Autodesk Fusion 360 part; units mm, degrees
note: some values were not read from the file. Set by a fixed rule: which face or edge a step refers to.
(part 3 of 4)
sketch "Sketch60" plane through (0, 0, 0) normal (0, -1, 0) x (1, 0, 0)
  arc A0 (-197.8622, -246.9544) -> (-202.8622, -246.9544) centre (-200.3622, -246.9544) ccw
  line L0 (-197.8622, -246.9544) -> (-197.8622, -256.8986)
  line L1 (-197.8622, -256.8986) -> (-177.6941, -256.8986)
  line L2 (-177.6941, -256.8986) -> (-177.6941, -247.1839)
  arc A1 (-172.6941, -247.1839) -> (-177.6941, -247.1839) centre (-175.1941, -247.1839) ccw
  line L3 (-172.6941, -247.1839) -> (-142.6941, -247.1839)
  line L4 (-142.6941, -247.1839) -> (-142.6941, -154.3986)
  arc A2 (-142.6941, -149.3986) -> (-142.6941, -154.3986) centre (-142.6941, -151.8986) ccw
  line L5 (-142.6941, -149.3986) -> (-132.6941, -149.3986)
  line L6 (-132.6941, -149.3986) -> (-132.6941, -119.3986)
  line L7 (-132.6941, -119.3986) -> (-142.6941, -119.3986)
  arc A3 (-142.6941, -114.3986) -> (-142.6941, -119.3986) centre (-142.6941, -116.8986) ccw
  line L8 (-142.6941, -114.3986) -> (-142.6941, -16.8986)
  arc A4 (-142.6941, -11.8986) -> (-142.6941, -16.8986) centre (-142.6941, -14.3986) ccw
  line L9 (-142.6941, -11.8986) -> (-132.6941, -11.8986)
  line L10 (-132.6941, -11.8986) -> (-132.6941, 18.1014)
  line L11 (-132.6941, 18.1014) -> (-142.6941, 18.1014)
  arc A5 (-142.6941, 23.1014) -> (-142.6941, 18.1014) centre (-142.6941, 20.6014) ccw
  line L12 (-142.6941, 23.1014) -> (-142.6941, 120.6018)
  arc A6 (-142.6941, 125.6009) -> (-142.6941, 120.6018) centre (-142.6471, 123.1014) ccw
  line L13 (-142.6941, 125.6009) -> (-142.6941, 125.6014)
  line L14 (-142.6941, 125.6014) -> (-132.6941, 125.6014)
  line L15 (-132.6941, 125.6014) -> (-132.6941, 155.5705)
  line L16 (-132.6941, 155.5705) -> (-142.6941, 155.5705)
  line L17 (-142.6941, 155.5705) -> (-142.6941, 155.6018)
  arc A7 (-142.6941, 160.6009) -> (-142.6941, 155.6018) centre (-142.6471, 158.1014) ccw
  line L18 (-142.6941, 160.6009) -> (-142.6941, 263.1014)
  line L19 (-142.6941, 263.1014) -> (-167.6941, 263.1014)
  arc A8 (-172.6941, 263.1014) -> (-167.6941, 263.1014) centre (-170.1941, 263.1014) ccw
  line L20 (-172.6941, 263.1014) -> (-172.6941, 273.1014)
  line L21 (-172.6941, 273.1014) -> (-202.6941, 273.1014)
  line L22 (-202.6941, 273.1014) -> (-202.6941, 263.1014)
  arc A9 (-207.6941, 263.1014) -> (-202.6941, 263.1014) centre (-205.1941, 263.1014) ccw
  line L23 (-207.6941, 263.1014) -> (-232.6941, 263.1014)
  line L24 (-232.6941, 263.1014) -> (-232.6941, 198.1014)
  line L25 (-232.6941, 198.1014) -> (-222.6941, 198.1014)
  arc A10 (-222.6941, 193.1014) -> (-222.6941, 198.1014) centre (-222.6941, 195.6014) ccw
  line L26 (-222.6941, 193.1014) -> (-222.6941, 183.1014)
  arc A11 (-222.6941, 178.1014) -> (-222.6941, 183.1014) centre (-222.6941, 180.6014) ccw
  line L27 (-222.6941, 178.1014) -> (-232.6941, 178.1014)
  line L28 (-232.6941, 178.1014) -> (-232.6941, 163.1014)
  line L29 (-232.6941, 163.1014) -> (-332.6941, 163.1014)
  line L30 (-332.6941, 163.1014) -> (-332.6941, 178.1014)
  line L31 (-332.6941, 178.1014) -> (-342.6941, 178.1014)
  arc A12 (-342.6941, 183.1014) -> (-342.6941, 178.1014) centre (-342.6941, 180.6014) ccw
  line L32 (-342.6941, 183.1014) -> (-342.6941, 193.1014)
  arc A13 (-342.6941, 198.1014) -> (-342.6941, 193.1014) centre (-342.6941, 195.6014) ccw
  line L33 (-342.6941, 198.1014) -> (-332.6941, 198.1014)
  line L34 (-332.6941, 198.1014) -> (-332.6941, 263.1014)
  line L35 (-332.6941, 263.1014) -> (-357.6941, 263.1014)
  arc A14 (-362.6941, 263.1014) -> (-357.6941, 263.1014) centre (-360.1941, 263.1014) ccw
  line L36 (-362.6941, 263.1014) -> (-362.6941, 273.1014)
  line L37 (-362.6941, 273.1014) -> (-392.6941, 273.1014)
  line L38 (-392.6941, 273.1014) -> (-392.6941, 263.1014)
  arc A15 (-397.6941, 263.1014) -> (-392.6941, 263.1014) centre (-395.1941, 263.1014) ccw
  line L39 (-397.6941, 263.1014) -> (-422.6941, 263.1014)
  line L40 (-422.6941, 263.1014) -> (-422.6941, 160.6014)
  arc A16 (-422.6941, 155.6014) -> (-422.6941, 160.6014) centre (-422.6941, 158.1014) ccw
  line L41 (-422.6941, 155.6014) -> (-432.6941, 155.6014)
  line L42 (-432.6941, 155.6014) -> (-432.6941, 125.6014)
  line L43 (-432.6941, 125.6014) -> (-422.8505, 125.6014)
  arc A17 (-422.6941, 120.6038) -> (-422.8505, 125.6014) centre (-422.7723, 123.1026) ccw
  line L44 (-422.6941, 120.6038) -> (-422.6941, 23.1014)
  arc A18 (-422.6941, 18.1014) -> (-422.6941, 23.1014) centre (-422.6941, 20.6014) ccw
  line L45 (-422.6941, 18.1014) -> (-432.6941, 18.1014)
  line L46 (-432.6941, 18.1014) -> (-432.6941, -11.8986)
  line L47 (-432.6941, -11.8986) -> (-422.6941, -11.8986)
  arc A19 (-422.6941, -16.8986) -> (-422.6941, -11.8986) centre (-422.6941, -14.3986) ccw
  line L48 (-422.6941, -16.8986) -> (-422.6941, -114.3986)
  arc A20 (-422.6941, -119.3986) -> (-422.6941, -114.3986) centre (-422.6941, -116.8986) ccw
  line L49 (-422.6941, -119.3986) -> (-432.6941, -119.3986)
  line L50 (-432.6941, -119.3986) -> (-432.6941, -149.3986)
  line L51 (-432.6941, -149.3986) -> (-422.6941, -149.3986)
  arc A21 (-422.6941, -154.3986) -> (-422.6941, -149.3986) centre (-422.6941, -151.8986) ccw
  line L52 (-422.6941, -154.3986) -> (-422.6941, -246.8986)
  line L53 (-422.6941, -246.8986) -> (-392.6941, -246.8986)
  arc A22 (-387.6941, -246.8986) -> (-392.6941, -246.8986) centre (-390.1941, -246.8986) ccw
  line L54 (-387.6941, -246.8986) -> (-387.6941, -256.8986)
  line L55 (-387.6941, -256.8986) -> (-367.8622, -256.8986)
  line L56 (-367.8622, -256.8986) -> (-367.8622, -246.9544)
  arc A23 (-362.8622, -246.9544) -> (-367.8622, -246.9544) centre (-365.3622, -246.9544) ccw
  line L57 (-362.8622, -246.9544) -> (-202.8622, -246.9544)
  line L58 (-365.1941, -66.8986) -> (-365.1941, 98.1014)
  line L59 (-365.1941, 98.1014) -> (-200.1941, 98.1014)
  line L60 (-200.1941, 98.1014) -> (-200.1941, -66.8986)
  line L61 (-200.1941, -66.8986) -> (-365.1941, -66.8986)
  line L62 (-406.2361, -111.2993) -> (-206.2361, -111.2993)
  line L63 (-206.2361, -111.2993) -> (-206.2361, -161.2993)
  line L64 (-206.2361, -161.2993) -> (-406.2361, -161.2993)
  line L65 (-406.2361, -161.2993) -> (-406.2361, -111.2993)
  dimension "d334" = 200
  dimension "d335" = 50
  constraint horizontal L62
  constraint vertical L63
  constraint horizontal L64
  constraint vertical L65
  measures "d334" distance of L62.start L62.end
  measures "d335" distance of L62.start L64.end
extrude "Extrude39" add sketch "Sketch60" along normal blind 8 separate body contours L62 L63 L64 L65 makes body 10
sketch "Sketch61" plane through (-206.2361, 0, 0) normal (1, 0, 0) x (0, 1, 0)
  line L0 (0, -161.2993) -> (0, -111.2993)
  line L1 (0, -111.2993) -> (-8, -111.2993)
  line L2 (-8, -111.2993) -> (-8, -161.2993)
  line L3 (-8, -161.2993) -> (0, -161.2993)
  line L4 (-68, -111.2993) -> (-8, -111.2993)
  line L5 (-8, -111.2993) -> (-8, -161.2993)
  line L6 (-8, -161.2993) -> (-68, -161.2993)
  line L7 (-73, -156.2993) -> (-73, -116.2993)
  arc A0 (-68, -111.2993) -> (-73, -116.2993) centre (-68, -116.2993) ccw
  arc A1 (-73, -156.2993) -> (-68, -161.2993) centre (-68, -156.2993) ccw
  dimension "d340" = 10
  dimension "d341" = 10
  constraint horizontal L4
  constraint vertical L5
  constraint horizontal L6
  constraint vertical L7
  constraint coincident L1.end L2.start
  constraint tangent L4 A0
  constraint tangent L7 A0
  constraint tangent L6 A1
  constraint tangent L7 A1
  measures "d340" diameter of A0
  measures "d341" diameter of A1
extrude "Extrude40" add sketch "Sketch61" against normal blind 10 separate body contours L2 L4 L5 L6 L7 A0 A1 makes body 11
sketch "Sketch62" plane through (0, 0, 0) normal (0, 1, 0) x (1, 0, 0)
sketch "Sketch63" plane through (-216.2361, 0, 0) normal (-1, 0, 0) x (0, -1, 0)
  arc A0 (73, -116.2993) -> (68, -111.2993) centre (68, -116.2993) ccw
  line L0 (68, -111.2993) -> (8, -111.2993)
  line L1 (8, -111.2993) -> (8, -161.2993)
  line L2 (8, -161.2993) -> (68, -161.2993)
  arc A1 (68, -161.2993) -> (73, -156.2993) centre (68, -156.2993) ccw
  line L3 (73, -156.2993) -> (73, -116.2993)
  circle A2 centre (170, -90) radius 18.5
  dimension "d351" = 37
  measures "d351" diameter of A2
extrude "Extrude41" add sketch "Sketch63" along normal blind 57 separate body contours A2 makes body 12
sketch "Sketch64" plane through (-216.2361, 0, 0) normal (1, 0, 0) x (0, 1, 0)
  circle A0 centre (-170, -90) radius 3
  circle A1 centre (-170, -90) radius 18.5
  dimension "d357" = 6
  constraint concentric A0 A1
  measures "d357" diameter of A0
extrude "Extrude42" add sketch "Sketch64" along normal blind 20 contours A0 bodies 12
sketch "Sketch65" plane through (0, 0, -111.2993) normal (0, 0, 1) x (-1, 0, 0)
  line L0 (206.2361, 0) -> (406.2361, 0)
  line L1 (406.2361, 0) -> (406.2361, 8)
  line L2 (406.2361, 8) -> (206.2361, 8)
  line L3 (206.2361, 8) -> (206.2361, 0)
  line L4 (538, -190) -> (498, -190)
  line L5 (498, -190) -> (498, -188)
  line L6 (498, -188) -> (538, -188)
  line L7 (538, -188) -> (538, -190)
  line L8 (500, -190) -> (498, -190)
  line L9 (498, -190) -> (498, -147)
  line L10 (498, -147) -> (500, -147)
  line L11 (500, -147) -> (500, -190)
  dimension "d360" = 40
  dimension "d361" = 2
  dimension "d362" = 2
  dimension "d363" = 43
  constraint horizontal L4
  constraint vertical L5
  constraint horizontal L6
  constraint vertical L7
  constraint horizontal L8
  constraint vertical L9
  constraint horizontal L10
  constraint vertical L11
  constraint coincident L4.end L5.start
  measures "d360" distance of L4.start L4.end
  measures "d361" distance of L4.start L6.end
  measures "d362" distance of L8.start L4.end
  measures "d363" distance of L8.start L10.end
extrude "Extrude43" add sketch "Sketch65" along normal blind 40 separate body contours L4 L6 L7 L11 | L4 L5 L6 L8 L9 L11 | L6 L9 L10 L11 makes body 13
sketch "Sketch66" plane through (0, 0, 0) normal (0, 0, 1) x (1, 0, 0)
sketch "Sketch67" plane through (0, 0, 0) normal (0, -1, 0) x (1, 0, 0)
move_body "Move6" bodies 13 to x (1, 0, 0) y (0, 1, 0) z (0, 0, 1) at (-242.0057, 0, -461.3258)
sketch "Sketch68" plane through (-740.0057, 0, 0) normal (1, 0, 0) x (0, 1, 0)
  line L0 (147, -572.6251) -> (190, -572.6251)
  line L1 (190, -572.6251) -> (190, -532.6251)
  line L2 (190, -532.6251) -> (147, -532.6251)
  line L3 (147, -532.6251) -> (147, -572.6251)
  line L4 (167, -532.6251) -> (190, -532.6251)
  line L5 (190, -532.6251) -> (190, -572.6251)
  line L6 (190, -572.6251) -> (167, -572.6251)
  arc A0 (167, -532.6251) -> (167, -572.6251) centre (167, -552.6251) ccw
  dimension "d366" = 43
  constraint horizontal L4
  constraint vertical L5
  constraint horizontal L6
  constraint tangent L4 A0
  constraint tangent L6 A0
  measures "d366" distance of L2.end L1.end
extrude "Extrude44" cut sketch "Sketch68" against normal blind 2 contours L0 L3 A0 | L2 L3 A0 bodies 13
sketch "Sketch69" plane through (-740.0057, 0, 0) normal (1, 0, 0) x (0, 1, 0)
  arc A0 (167, -532.6251) -> (167, -572.6251) centre (167, -552.6251) ccw
  line L0 (167, -572.6251) -> (190, -572.6251)
  line L1 (190, -572.6251) -> (190, -532.6251)
  line L2 (190, -532.6251) -> (167, -532.6251)
  circle A1 centre (168.5, -552.6251) radius 3
  dimension "d370" = 6
  measures "d370" diameter of A1
extrude "Extrude45" cut sketch "Sketch69" against normal blind 2 contours A1 bodies 13
sketch "Sketch70" plane through (-742.0057, 0, 0) normal (-1, 0, 0) x (0, -1, 0)
  circle A0 centre (-168.5, -552.6251) radius 3
move_body "Move7" bodies 12 to x (1, 0, 0) y (0, 1, 0) z (0, 0, 1) at (0, -222.4188, 95.0256)
move_body "Move8" bodies 12 to x (1, 0, 0) y (0, 1, 0) z (0, 0, 1) at (-545, 614.0985, -612.4606)
move_body "Move9" bodies 12 to x (1, 0, 0) y (0, 0.965926, 0.258819) z (0, -0.258819, 0.965926) at (19.4785, -202.815, -23.1256)
move_body "Move10" bodies 12 13 to x (1, 0, 0) y (0, 1, 0) z (0, 0, 1) at (392.4146, -197.9462, 415.5182)
sketch "Sketch71" plane through (-347.591, 0, 0) normal (1, 0, 0) x (0, 1, 0)
  circle A0 centre (-29.4462, -137.1069) radius 3
  arc A1 (-30.9462, -117.1069) -> (-30.9462, -157.1069) centre (-30.9462, -137.1069) ccw
  line L0 (-30.9462, -157.1069) -> (-7.9462, -157.1069)
  line L1 (-7.9462, -157.1069) -> (-7.9462, -117.1069)
  line L2 (-7.9462, -117.1069) -> (-30.9462, -117.1069)
  circle A2 centre (-29.4462, -137.1069) radius 3
  dimension "d373" = 6
  constraint concentric A0 A2
  measures "d373" diameter of A2
extrude "Extrude46" add 1 faces at (-329.343, -30.6538, -136.491) along direction (1, 0, 0) blind 120 separate body on bodies 12 makes body 14
sketch "Sketch72" plane through (0, 0, 0) normal (0, 1, 0) x (1, 0, 0)
extrude "Extrude47" add 1 faces at (-209.343, -30.6538, -136.491) along direction (1, 0, 0) blind 10 on bodies 14 bodies 14
sketch "Sketch73" plane through (-206.2361, 0, 0) normal (1, 0, 0) x (0, 1, 0)
  arc A0 (-68, -111.2993) -> (-73, -116.2993) centre (-68, -116.2993) ccw
  line L0 (-73, -116.2993) -> (-73, -156.2993)
  arc A1 (-73, -156.2993) -> (-68, -161.2993) centre (-68, -156.2993) ccw
  line L1 (-68, -161.2993) -> (-8, -161.2993)
  line L2 (-8, -161.2993) -> (-8, -111.2993)
  line L3 (-8, -111.2993) -> (-68, -111.2993)
  circle A2 centre (-29.4462, -137.1069) radius 3.25
  circle A3 centre (-29.4462, -137.1069) radius 3
  dimension "d379" = 6.5
  constraint concentric A2 A3
  measures "d379" diameter of A2
extrude "Extrude48" cut sketch "Sketch73" against normal through all contours A3 bodies 11
sketch "Sketch74" plane through (-206.2361, 0, 0) normal (1, 0, 0) x (0, 1, 0)
sketch "Sketch75" plane through (-216.2361, 0, 0) normal (-1, 0, 0) x (0, -1, 0)
sketch "Sketch76" plane through (-206.2361, 0, 0) normal (1, 0, 0) x (0, 1, 0)
sketch "Sketch77" plane through (-199.343, 0, 0) normal (1, 0, 0) x (0, 1, 0)
sketch "Sketch78" plane through (-216.2361, 0, 0) normal (-1, 0, 0) x (0, -1, 0)
sketch "Sketch79" plane through (-216.2361, -40.5, -136.2993) normal (-1, 0, 0) x (0, -1, 0)
sketch "Sketch80" plane through (-206.2361, 0, 0) normal (1, 0, 0) x (0, 1, 0)
  line L0 (-35, -130) -> (-21.0963, -130)
  line L1 (-21.0963, -130) -> (-21.0963, -147.7881)
  line L2 (-21.0963, -147.7881) -> (-35, -147.7881)
  line L3 (-35, -147.7881) -> (-35, -130)
  constraint horizontal L0
  constraint vertical L1
  constraint horizontal L2
  constraint vertical L3
extrude "Extrude50" add sketch "Sketch80" against normal blind 10 bodies 11
sketch "Sketch81" plane through (-206.2361, 0, 0) normal (1, 0, 0) x (0, 1, 0)
  line L0 (-32.4193, -136.2247) -> (-26.4193, -136.2247)
  circle A0 centre (-29.4193, -136.2247) radius 3.25
  dimension "d387" = 6.5
  constraint horizontal L0
  constraint midpoint L0 A0.centre
  measures "d387" diameter of A0
extrude "Extrude51" cut sketch "Sketch81" against normal blind 10 bodies 11
move_face "MoveFace1" by (1, 0, 0) 1 faces at (-199.343, -30.6538, -136.491) on bodies 14
move_face "MoveFace2" by (0, 0, 1.4691) 1 faces at (-329.343, -28.1848, -137.4483) on bodies 14
move_body "Move11" bodies 14 to x (1, 0, 0) y (0, 1, 0) z (0, 0, 1) at (0, 0, 0.5)
move_body "Move12" bodies 14 to x (1, 0, 0) y (0, 1, 0) z (0, 0, 1) at (0, 0, 0.25)
move_body "Move13" bodies 12 to x (1, 0, 0) y (0, 1, 0) z (0, 0, 1) at (0, 0, 0.75)
move_body "Move14" bodies 13 to x (1, 0, 0) y (0, 1, 0) z (0, 0, 1) at (0, 0, 0.75)
sketch "Sketch83" plane through (0, 0, 0) normal (0, 0, 1) x (1, 0, 0)
sketch "Sketch84" plane through (-206.2361, 0, 0) normal (1, 0, 0) x (0, 1, 0)
sketch "Sketch85" plane through (-206.2361, 0, 0) normal (1, 0, 0) x (0, 1, 0)
  line L0 (-53.5087, -133.0971) -> (-40.8265, -133.0836)
  line L1 (-53.5087, -139.0701) -> (-40.8265, -139.0836)
  arc A0 (-52.9462, -133.0965) -> (-52.9462, -139.0707) centre (-53.2243, -136.0836) ccw
  arc A1 (-40.8265, -139.0836) -> (-40.8265, -133.0836) centre (-40.8233, -136.0836) ccw
  dimension "d394" = 6
  dimension "d395" = 6
  constraint coincident L0.start A0
  constraint tangent L0 A1
  constraint coincident L1.start A0
  constraint tangent L1 A1
  constraint coincident L1 A0.end
  constraint coincident L0 A0.start
  measures "d394" diameter of A1
  measures "d395" diameter of A0
sketch "Sketch86" plane through (-216.2361, 0, 0) normal (-1, 0, 0) x (0, -1, 0)
sketch "Sketch87" plane through (-216.2361, 0, 0) normal (-1, 0, 0) x (0, -1, 0)
  circle A0 centre (29.4193, -136.2196) radius 6.5
  circle A1 centre (29.4193, -136.2196) radius 3
  dimension "d398" = 13
  constraint concentric A0 A1
  measures "d398" diameter of A0
extrude "Extrude52" cut sketch "Sketch85" against normal blind 10 contours L0 L1 A0 A1 bodies 11
extrude "Extrude53" add sketch "Sketch87" along normal blind 90 bodies 14
sketch "Sketch88" plane through (0, -73, 0) normal (0, -1, 0) x (1, 0, 0)
  line L0 (-206.2361, -156.2993) -> (-206.2361, -116.2993)
  line L1 (-206.2361, -116.2993) -> (-216.2361, -116.2993)
  line L2 (-216.2361, -116.2993) -> (-216.2361, -156.2993)
  line L3 (-216.2361, -156.2993) -> (-206.2361, -156.2993)
  circle A0 centre (-211.2361, -136.2993) radius 3
  dimension "d403" = 6
  measures "d403" diameter of A0
extrude "Extrude54" cut sketch "Sketch88" against normal blind 10 contours A0 bodies 11
copy_body "CopyPasteBodies4" bodies 11 makes body 15
move_body "Move15" bodies 15 to x (1, 0, 0) y (0, 1, 0) z (0, 0, 1) at (-91, 0, 0)
move_body "Move16" bodies 15 to x (1, 0, 0) y (0, 1, 0) z (0, 0, 1) at (-10, 0, 0)
sketch "Sketch89" plane through (0, -73, 0) normal (0, -1, 0) x (1, 0, 0)
  circle A0 centre (-312.2361, -136.2993) radius 3
  line L0 (-307.2361, -156.2993) -> (-307.2361, -116.2993)
  line L1 (-307.2361, -116.2993) -> (-317.2361, -116.2993)
  line L2 (-317.2361, -116.2993) -> (-317.2361, -156.2993)
  line L3 (-317.2361, -156.2993) -> (-307.2361, -156.2993)
  line L4 (-317.2361, -116.2993) -> (-307.2361, -116.2993)
  line L5 (-307.2361, -116.2993) -> (-307.2361, -156.2993)
  line L6 (-307.2361, -156.2993) -> (-317.2361, -156.2993)
  line L7 (-317.2361, -156.2993) -> (-317.2361, -116.2993)
  line L8 (-312.2361, -116.2993) -> (-312.2361, -156.2993)
  circle A1 centre (-312.2361, -123.7993) radius 2
  circle A2 centre (-312.2361, -148.7993) radius 2
  dimension "d406" = 10
  dimension "d407" = 40
  dimension "d410" = 4
  dimension "d411" = 4
  constraint horizontal L4
  constraint vertical L5
  constraint horizontal L6
  constraint vertical L7
  constraint coincident L1.end L2.start
  constraint midpoint L4 L8.start
  constraint midpoint L6 L8.end
  constraint coincident L8 A1.centre
  constraint coincident L8 A2.centre
  measures "d406" distance of L1.end L0.end
  measures "d407" distance of L1.end L2.end
  measures "d410" diameter of A1
  measures "d411" diameter of A2
extrude "Extrude55" add sketch "Sketch89" along normal blind 3 separate body contours A0 L0 L1 L3 L4 L5 L6 L8 A1 A2 | A0 L1 L2 L3 L4 L6 L7 L8 A1 A2 makes body 16
copy_body "CopyPasteBodies5" bodies 16 makes body 17
move_body "Move17" bodies 17 to x (1, 0, 0) y (0, 1, 0) z (0, 0, 1) at (92, 0, 0)
move_body "Move18" bodies 17 to x (1, 0, 0) y (0, 1, 0) z (0, 0, 1) at (9, 0, 0)
sketch "Sketch90" plane through (-216.2361, 0, 0) normal (-1, 0, 0) x (0, -1, 0)
sketch "Sketch91" plane through (-216.2361, 0, 0) normal (-1, 0, 0) x (0, -1, 0)
  circle A0 centre (49.2242, -136.0566) radius 3
  dimension "d416" = 6
  measures "d416" diameter of A0
sketch "Sketch92" plane through (-216.2361, 0, 0) normal (-1, 0, 0) x (0, -1, 0)
surface "Extrude56" add extruded along (-1, 0, 0) between 0 and -15 path "Sketch91" along A0 separate body makes body 18
sketch "Sketch93" plane through (-206.2361, 0, 0) normal (1, 0, 0) x (0, 1, 0)
  circle A0 centre (-49.2242, -136.0566) radius 3
  circle A1 centre (-49.2242, -136.0566) radius 3
  dimension "d424" = 6
  constraint concentric A0 A1
  measures "d424" diameter of A0
extrude "Extrude57" cut sketch "Sketch93" against normal blind 110 bodies 15
delete_face "SurfaceDeleteFace1" leaving the opening 1 faces at (-206.2361, -51.9886, -134.8913) on bodies 18
sketch "Sketch94" plane through (-206.2361, 0, 0) normal (1, 0, 0) x (0, 1, 0)
  circle A0 centre (-29.4193, -136.2196) radius 6.5
  circle A1 centre (-29.4193, -136.2196) radius 3
  circle A2 centre (-48.4163, -135.8821) radius 12.5
  circle A3 centre (-48.4163, -135.8821) radius 3
  dimension "d427" = 13
  dimension "d428" = 25
  dimension "d429" = 6
  constraint concentric A0 A1
  constraint tangent A0 A2
  constraint concentric A2 A3
  measures "d427" diameter of A0
  measures "d428" diameter of A2
  measures "d429" diameter of A3
extrude "Extrude58" add sketch "Sketch94" along normal blind 10 and the other way blind 120 separate body contours A3 makes body 19
sketch "Sketch95" plane through (-196.2361, 0, 0) normal (1, 0, 0) x (0, 1, 0)
  circle A0 centre (-48.4163, -135.8821) radius 3
  circle A1 centre (-48.4163, -135.8821) radius 12.5
  dimension "d434" = 25
  constraint concentric A0 A1
  measures "d434" diameter of A1
extrude "Extrude59" add sketch "Sketch95" against normal blind 10 separate body contours A0 | A1 makes body 20
move_face "MoveFace3" to x (1, 0, 0) y (0, 1, 0) z (0, 0, 1) at (10, 0, 0) 1 faces at (-202.9028, -35.9318, -136.5052) on bodies 20
move_body "Move19" bodies 20 to x (1, 0, 0) y (0, 1, 0) z (0, 0, 1) at (-20, 0, 0)
move_face "MoveFace4" to x (1, 0, 0) y (0, 1, 0) z (0, 0, 1) at (-80, 0, 0) 1 faces at (-222.9028, -35.9318, -136.5052) on bodies 20
copy_body "CopyPasteBodies6" bodies 20 makes body 21
move_body "Move20" bodies 21 to x (1, 0, 0) y (0, 1, 0) z (0, 0, 1) at (-80, 0, 0)
copy_body "CopyPasteBodies7" bodies 20 makes body 22
move_body "Move21" bodies 22 to x (1, 0, 0) y (0, 1, 0) z (0, 0, 1) at (-40, 0, 0)
copy_body "CopyPasteBodies8" bodies 20 makes body 23
move_body "Move22" bodies 23 to x (1, 0, 0) y (0, 1, 0) z (0, 0, 1) at (-20, 0, 0)
copy_body "CopyPasteBodies9" bodies 22 makes body 24
move_body "Move23" bodies 24 to x (1, 0, 0) y (0, 1, 0) z (0, 0, 1) at (-20, 0, 0)
move_body "Move24" bodies 9 to x (-0.707107, -0.707107, 0) y (0.707107, -0.707107, 0) z (0, 0, 1) at (-660.8733, -493.7427, 0)
sketch "Sketch96" plane through (0, -10, 0) normal (0, -1, 0) x (1, 0, 0)
  line L0 (-200.1941, -66.8986) -> (-365.1941, -66.8986)
  line L1 (-365.1941, -66.8986) -> (-365.1941, 98.1014)
  line L2 (-365.1941, 98.1014) -> (-200.1941, 98.1014)
  line L3 (-200.1941, 98.1014) -> (-200.1941, -66.8986)
  line L4 (-142.6941, 135.6014) -> (-422.6941, 135.6014)
  line L5 (-422.6941, 135.6014) -> (-422.6941, -104.3986)
  line L6 (-422.6941, -104.3986) -> (-142.6941, -104.3986)
  line L7 (-142.6941, -104.3986) -> (-142.6941, 135.6014)
  line L8 (-365.1941, 98.1014) -> (-200.1941, 98.1014)
  line L9 (-200.1941, 98.1014) -> (-200.1941, -66.8986)
  line L10 (-200.1941, -66.8986) -> (-365.1941, -66.8986)
  line L11 (-365.1941, -66.8986) -> (-365.1941, 98.1014)
  line L12 (-382.6941, 115.6014) -> (-182.6941, 115.6014)
  line L13 (-182.6941, 115.6014) -> (-182.6941, -84.3986)
  line L14 (-182.6941, -84.3986) -> (-382.6941, -84.3986)
  line L15 (-382.6941, -84.3986) -> (-382.6941, 115.6014)
  dimension "d438" = 165
  dimension "d439" = 165
  dimension "d440" = 200
  dimension "d441" = 200
  constraint horizontal L8
  constraint vertical L9
  constraint horizontal L10
  constraint vertical L11
  constraint coincident L1.end L2.start
  constraint horizontal L12
  constraint vertical L13
  constraint horizontal L14
  constraint vertical L15
  measures "d438" distance of L1.end L2.end
  measures "d439" distance of L1.end L0.end
  measures "d440" distance of L12.start L12.end
  measures "d441" distance of L12.start L14.end
extrude "Extrude60" add sketch "Sketch96" along normal blind 3 separate body contours L12 L13 L14 L15 makes body 25
sketch "Sketch97" plane through (0, -13, 0) normal (0, -1, 0) x (1, 0, 0)
  line L0 (-200.1941, -66.8986) -> (-365.1941, -66.8986)
  line L1 (-365.1941, -66.8986) -> (-365.1941, 98.1014)
  line L2 (-365.1941, 98.1014) -> (-200.1941, 98.1014)
  line L3 (-200.1941, 98.1014) -> (-200.1941, -66.8986)
  line L4 (-382.6941, -84.3986) -> (-182.6941, -84.3986)
  line L5 (-182.6941, -84.3986) -> (-182.6941, 115.6014)
  line L6 (-182.6941, 115.6014) -> (-382.6941, 115.6014)
  line L7 (-382.6941, 115.6014) -> (-382.6941, -84.3986)
  line L8 (-376.8614, -55.2314) -> (-353.5268, -78.5659)
  line L9 (-353.5268, -78.5659) -> (-360.5979, -85.637)
  line L10 (-360.5979, -85.637) -> (-383.9324, -62.3024)
  line L11 (-383.9324, -62.3024) -> (-376.8614, -55.2314)
  line L12 (-181.4558, 93.5052) -> (-188.5268, 86.4341)
  line L13 (-211.8614, 109.7686) -> (-204.7903, 116.8397)
  line L14 (-188.5268, 86.4341) -> (-211.8614, 109.7686)
  line L15 (-204.7903, 116.8397) -> (-181.4558, 93.5052)
  line L16 (-353.5268, 109.7686) -> (-376.8614, 86.4341)
  line L17 (-383.9324, 93.5052) -> (-360.5979, 116.8397)
  line L18 (-360.5979, 116.8397) -> (-353.5268, 109.7686)
  line L19 (-376.8614, 86.4341) -> (-383.9324, 93.5052)
  line L20 (-210.8007, -77.5052) -> (-189.5875, -56.292)
  line L21 (-189.5875, -56.292) -> (-182.5164, -63.3631)
  line L22 (-182.5164, -63.3631) -> (-203.7296, -84.5763)
  line L23 (-203.7296, -84.5763) -> (-210.8007, -77.5052)
  dimension "d444" = 33
  dimension "d445" = 10
  dimension "d446" = 33
  dimension "d447" = 10
  dimension "d448" = 33
  dimension "d449" = 10
  dimension "d450" = 30
  dimension "d451" = 10
  constraint midpoint L2.end L14
  constraint midpoint L0.end L8
  constraint midpoint L1.end L16
  constraint midpoint L0.start L20
  measures "d444" distance of L8.start L8.end
  measures "d445" distance of L8.start L10.end
  measures "d446" distance of L12.start L13.end
  measures "d447" distance of L13.end L13.start
  measures "d448" distance of L16.end L16.start
  measures "d449" distance of L16.start L17.end
  measures "d450" distance of L20.start L20.end
  measures "d451" distance of L20.start L22.end
extrude "Extrude61" add sketch "Sketch97" along normal blind 25 separate body contours L4 L5 L20 L21 L22 L23 | L4 L7 L8 L9 L10 L11 | L5 L6 L12 L13 L14 L15 | L6 L7 L16 L17 L18 L19 makes body 26 at (-196.305, -29.6667, 94.2123) makes body 27 at (-203.7296, -21.3333, -70.4342) makes body 28 at (-361.305, -29.6667, 101.9904) makes body 29 at (-369.0832, -21.3333, -63.0096)
sketch "Sketch98" plane through (0, 0, 0) normal (0, -1, 0) x (1, 0, 0)
  circle A0 centre (-282.6941, 15.6014) radius 82.5
  line L0 (-392.6941, 136.1014) -> (-172.6941, 136.1014)
  line L1 (-152.6941, 116.1014) -> (-152.6941, -83.8986)
  line L2 (-172.6941, -103.8986) -> (-392.6941, -103.8986)
  line L3 (-412.6941, -83.8986) -> (-412.6941, 116.1014)
  line L4 (-392.6941, 136.1014) -> (-412.6941, 116.1014)
  line L5 (-172.6941, 136.1014) -> (-152.6941, 116.1014)
  line L6 (-412.6941, -83.8986) -> (-392.6941, -103.8986)
  line L7 (-172.6941, -103.8986) -> (-152.6941, -83.8986)
  point P0 (-412.6941, 136.1014)
  point P1 (-152.6941, 136.1014)
  point P2 (-152.6941, -103.8986)
  point P3 (-412.6941, -103.8986)
  point P4 (-142.6941, 18.1014)
  dimension "d454" = 260
  dimension "d455" = 240
  dimension "d456" = 20
  dimension "d457" = 20
  dimension "d458" = 20
  dimension "d459" = 20
  dimension "d460" = 20
  dimension "d461" = 20
  dimension "d462" = 20
  dimension "d463" = 20
  constraint horizontal L0
  constraint vertical L1
  constraint horizontal L2
  constraint vertical L3
  constraint coincident P0 L0
  constraint coincident P0 L3
  constraint coincident P1 L0
  constraint coincident P1 L1
  constraint coincident P3 L3
  constraint coincident P3 L2
  constraint coincident P2 L2
  constraint coincident P2 L1
  measures "d454" distance of P0 P1
  measures "d455" distance of P0 P3
  measures "d456" distance of P0 L0.start
  measures "d457" distance of P0 L3.end
  measures "d458" distance of P1 L0.end
  measures "d459" distance of P1 L1.start
  measures "d460" distance of P3 L3.start
  measures "d461" distance of P3 L2.end
  measures "d462" distance of P2 L2.start
  measures "d463" distance of P2 L1.end
extrude "Extrude62" add sketch "Sketch98" along normal blind 3 separate body makes body 30
sketch "Sketch99" plane through (-132.6941, 0, 0) normal (1, 0, 0) x (0, 1, 0)
  circle A0 centre (-25, -180) radius 4
  circle A1 centre (-50, 175) radius 4
  circle A2 centre (-25, 170) radius 4
  circle A3 centre (-50, -175) radius 4
  circle A4 centre (-75, 180) radius 4
  circle A5 centre (-75, -170) radius 4
  line L0 (0, 130.6014) -> (0, 150.6014)
  arc A6 (0, 155.6014) -> (0, 150.6014) centre (0, 153.1014) ccw
  line L1 (0, 155.6014) -> (10, 155.6014)
  line L2 (10, 155.6014) -> (10, 273.6512)
  line L3 (10, 273.6512) -> (-30, 273.6512)
  line L4 (-30, 273.6512) -> (-30, 263.6512)
  arc A7 (-35, 263.6512) -> (-30, 263.6512) centre (-32.5, 263.6512) ccw
  line L5 (-35, 263.6512) -> (-55, 263.6512)
  arc A8 (-60, 263.6512) -> (-55, 263.6512) centre (-57.5, 263.6512) ccw
  line L6 (-60, 263.6512) -> (-60, 273.6512)
  line L7 (-60, 273.6512) -> (-100, 273.6512)
  line L8 (-100, 273.6512) -> (-100, -256.3488)
  line L9 (-100, -256.3488) -> (-60, -256.3488)
  line L10 (-60, -256.3488) -> (-60, -246.3488)
  arc A9 (-55, -246.3488) -> (-60, -246.3488) centre (-57.5, -246.3488) ccw
  line L11 (-55, -246.3488) -> (-35, -246.3488)
  arc A10 (-30, -246.3488) -> (-35, -246.3488) centre (-32.5, -246.3488) ccw
  line L12 (-30, -246.3488) -> (-30, -256.3488)
  line L13 (-30, -256.3488) -> (10, -256.3488)
  line L14 (10, -256.3488) -> (10, -149.3986)
  line L15 (10, -149.3986) -> (0, -149.3986)
  arc A11 (0, -144.3986) -> (0, -149.3986) centre (0, -146.8986) ccw
  line L16 (0, -144.3986) -> (0, -124.3986)
  arc A12 (0, -119.3986) -> (0, -124.3986) centre (0, -121.8986) ccw
  line L17 (0, -119.3986) -> (10, -119.3986)
  line L18 (10, -119.3986) -> (10, -11.8986)
  line L19 (10, -11.8986) -> (0, -11.8986)
  arc A13 (0, -6.8986) -> (0, -11.8986) centre (0, -9.3986) ccw
  line L20 (0, -6.8986) -> (0, 13.1014)
  arc A14 (0, 18.1014) -> (0, 13.1014) centre (0, 15.6014) ccw
  line L21 (0, 18.1014) -> (10, 18.1014)
  line L22 (10, 18.1014) -> (10, 125.6014)
  line L23 (10, 125.6014) -> (0, 125.6014)
  arc A15 (0, 130.6014) -> (0, 125.6014) centre (0, 128.1014) ccw
  circle A16 centre (-75, 160) radius 4
  circle A17 centre (-50, 155) radius 4
  circle A18 centre (-25, 150) radius 4
  circle A19 centre (-75, 140) radius 4
  circle A20 centre (-50, 135) radius 4
  circle A21 centre (-25, 130) radius 4
  circle A22 centre (-75, 120) radius 4
  circle A23 centre (-50, 115) radius 4
  circle A24 centre (-25, 110) radius 4
  dimension "d468" = 20
  dimension "d469" = 20
  dimension "d470" = 8
  dimension "d471" = 8
  dimension "d472" = 8
  dimension "d473" = 8
  dimension "d474" = 8
  dimension "d475" = 8
  dimension "d476" = 8
  dimension "d477" = 8
  dimension "d478" = 8
  measures "d468" distance of A4.centre A16.centre
  measures "d469" distance of A1.centre A17.centre
  measures "d470" diameter of A16
  measures "d471" diameter of A17
  measures "d472" diameter of A18
  measures "d473" diameter of A19
  measures "d474" diameter of A20
  measures "d475" diameter of A21
  measures "d476" diameter of A22
  measures "d477" diameter of A23
  measures "d478" diameter of A24
extrude "Extrude63" cut sketch "Sketch99" against normal blind 10 contours A16 | A17 | A18 | A19 | A20 | A21 | A22 | A23 | A24 bodies 2
sketch "Sketch100" plane through (-132.6941, 0, 0) normal (1, 0, 0) x (0, 1, 0)
  circle A0 centre (-75, 120) radius 4
  circle A1 centre (-25, 150) radius 4
  circle A2 centre (-50, 155) radius 4
  circle A3 centre (-25, 130) radius 4
  circle A4 centre (-50, 115) radius 4
  circle A5 centre (-75, 140) radius 4
  circle A6 centre (-75, 160) radius 4
  circle A7 centre (-50, 135) radius 4
  circle A8 centre (-25, 110) radius 4
  circle A9 centre (-25, -180) radius 4
  circle A10 centre (-50, 175) radius 4
  circle A11 centre (-25, 170) radius 4
  circle A12 centre (-50, -175) radius 4
  circle A13 centre (-75, 180) radius 4
  circle A14 centre (-75, -170) radius 4
  line L0 (0, 130.6014) -> (0, 150.6014)
  arc A15 (0, 155.6014) -> (0, 150.6014) centre (0, 153.1014) ccw
  line L1 (0, 155.6014) -> (10, 155.6014)
  line L2 (10, 155.6014) -> (10, 273.6512)
  line L3 (10, 273.6512) -> (-30, 273.6512)
  line L4 (-30, 273.6512) -> (-30, 263.6512)
  arc A16 (-35, 263.6512) -> (-30, 263.6512) centre (-32.5, 263.6512) ccw
  line L5 (-35, 263.6512) -> (-55, 263.6512)
  arc A17 (-60, 263.6512) -> (-55, 263.6512) centre (-57.5, 263.6512) ccw
  line L6 (-60, 263.6512) -> (-60, 273.6512)
  line L7 (-60, 273.6512) -> (-100, 273.6512)
  line L8 (-100, 273.6512) -> (-100, -256.3488)
  line L9 (-100, -256.3488) -> (-60, -256.3488)
  line L10 (-60, -256.3488) -> (-60, -246.3488)
  arc A18 (-55, -246.3488) -> (-60, -246.3488) centre (-57.5, -246.3488) ccw
  line L11 (-55, -246.3488) -> (-35, -246.3488)
  arc A19 (-30, -246.3488) -> (-35, -246.3488) centre (-32.5, -246.3488) ccw
  line L12 (-30, -246.3488) -> (-30, -256.3488)
  line L13 (-30, -256.3488) -> (10, -256.3488)
  line L14 (10, -256.3488) -> (10, -149.3986)
  line L15 (10, -149.3986) -> (0, -149.3986)
  arc A20 (0, -144.3986) -> (0, -149.3986) centre (0, -146.8986) ccw
  line L16 (0, -144.3986) -> (0, -124.3986)
  arc A21 (0, -119.3986) -> (0, -124.3986) centre (0, -121.8986) ccw
  line L17 (0, -119.3986) -> (10, -119.3986)
  line L18 (10, -119.3986) -> (10, -11.8986)
  line L19 (10, -11.8986) -> (0, -11.8986)
  arc A22 (0, -6.8986) -> (0, -11.8986) centre (0, -9.3986) ccw
  line L20 (0, -6.8986) -> (0, 13.1014)
  arc A23 (0, 18.1014) -> (0, 13.1014) centre (0, 15.6014) ccw
  line L21 (0, 18.1014) -> (10, 18.1014)
  line L22 (10, 18.1014) -> (10, 125.6014)
  line L23 (10, 125.6014) -> (0, 125.6014)
  arc A24 (0, 130.6014) -> (0, 125.6014) centre (0, 128.1014) ccw
  circle A25 centre (-75, 100) radius 4
  circle A26 centre (-50, 95) radius 4
  circle A27 centre (-25, 90) radius 4
  circle A28 centre (-75, 80) radius 4
  circle A29 centre (-50, 75) radius 4
  circle A30 centre (-25, 70) radius 4
  dimension "d481" = 8
  dimension "d482" = 8
  dimension "d483" = 8
  dimension "d484" = 8
  dimension "d485" = 8
  dimension "d486" = 8
  measures "d481" diameter of A25
  measures "d482" diameter of A26
  measures "d483" diameter of A27
  measures "d484" diameter of A28
  measures "d485" diameter of A29
  measures "d486" diameter of A30
extrude "Extrude64" cut sketch "Sketch100" against normal blind 10 contours A25 | A26 | A27 | A28 | A29 | A30 bodies 2
sketch "Sketch101" plane through (-132.6941, 0, 0) normal (1, 0, 0) x (0, 1, 0)
  circle A0 centre (-75, 80) radius 4
  circle A1 centre (-75, 100) radius 4
  circle A2 centre (-50, 75) radius 4
  circle A3 centre (-25, 90) radius 4
  circle A4 centre (-50, 95) radius 4
  circle A5 centre (-25, 70) radius 4
  circle A6 centre (-75, 120) radius 4
  circle A7 centre (-25, 150) radius 4
  circle A8 centre (-50, 155) radius 4
  circle A9 centre (-25, 130) radius 4
  circle A10 centre (-50, 115) radius 4
  circle A11 centre (-75, 140) radius 4
  circle A12 centre (-75, 160) radius 4
  circle A13 centre (-50, 135) radius 4
  circle A14 centre (-25, 110) radius 4
  circle A15 centre (-25, -180) radius 4
  circle A16 centre (-50, 175) radius 4
  circle A17 centre (-25, 170) radius 4
  circle A18 centre (-50, -175) radius 4
  circle A19 centre (-75, 180) radius 4
  circle A20 centre (-75, -170) radius 4
  line L0 (0, 130.6014) -> (0, 150.6014)
  arc A21 (0, 155.6014) -> (0, 150.6014) centre (0, 153.1014) ccw
  line L1 (0, 155.6014) -> (10, 155.6014)
  line L2 (10, 155.6014) -> (10, 273.6512)
  line L3 (10, 273.6512) -> (-30, 273.6512)
  line L4 (-30, 273.6512) -> (-30, 263.6512)
  arc A22 (-35, 263.6512) -> (-30, 263.6512) centre (-32.5, 263.6512) ccw
  line L5 (-35, 263.6512) -> (-55, 263.6512)
  arc A23 (-60, 263.6512) -> (-55, 263.6512) centre (-57.5, 263.6512) ccw
  line L6 (-60, 263.6512) -> (-60, 273.6512)
  line L7 (-60, 273.6512) -> (-100, 273.6512)
  line L8 (-100, 273.6512) -> (-100, -256.3488)
  line L9 (-100, -256.3488) -> (-60, -256.3488)
  line L10 (-60, -256.3488) -> (-60, -246.3488)
  arc A24 (-55, -246.3488) -> (-60, -246.3488) centre (-57.5, -246.3488) ccw
  line L11 (-55, -246.3488) -> (-35, -246.3488)
  arc A25 (-30, -246.3488) -> (-35, -246.3488) centre (-32.5, -246.3488) ccw
  line L12 (-30, -246.3488) -> (-30, -256.3488)
  line L13 (-30, -256.3488) -> (10, -256.3488)
  line L14 (10, -256.3488) -> (10, -149.3986)
  line L15 (10, -149.3986) -> (0, -149.3986)
  arc A26 (0, -144.3986) -> (0, -149.3986) centre (0, -146.8986) ccw
  line L16 (0, -144.3986) -> (0, -124.3986)
  arc A27 (0, -119.3986) -> (0, -124.3986) centre (0, -121.8986) ccw
  line L17 (0, -119.3986) -> (10, -119.3986)
  line L18 (10, -119.3986) -> (10, -11.8986)
  line L19 (10, -11.8986) -> (0, -11.8986)
  arc A28 (0, -6.8986) -> (0, -11.8986) centre (0, -9.3986) ccw
  line L20 (0, -6.8986) -> (0, 13.1014)
  arc A29 (0, 18.1014) -> (0, 13.1014) centre (0, 15.6014) ccw
  line L21 (0, 18.1014) -> (10, 18.1014)
  line L22 (10, 18.1014) -> (10, 125.6014)
  line L23 (10, 125.6014) -> (0, 125.6014)
  arc A30 (0, 130.6014) -> (0, 125.6014) centre (0, 128.1014) ccw
  circle A31 centre (-75, -150) radius 4
  circle A32 centre (-50, -155) radius 4
  circle A33 centre (-25, -160) radius 4
  circle A34 centre (-75, -130.3823) radius 4
  circle A35 centre (-50.7025, -135.281) radius 4
  circle A36 centre (-25, -140) radius 4
  circle A37 centre (-75, -110) radius 4
  circle A38 centre (-50, -115) radius 4
  circle A39 centre (-25, -120) radius 4
  circle A40 centre (-75, -90) radius 4
  circle A41 centre (-50, -95) radius 4
  circle A42 centre (-25, -100) radius 4
  circle A43 centre (-75, -70) radius 4
  circle A44 centre (-50, -75) radius 4
  circle A45 centre (-25, -80) radius 4
  dimension "d489" = 8
  dimension "d490" = 8
  dimension "d491" = 8
  dimension "d492" = 8
  dimension "d493" = 8
  dimension "d494" = 8
  dimension "d495" = 8
  dimension "d496" = 8
  dimension "d497" = 8
  dimension "d498" = 8
  dimension "d499" = 8
  dimension "d500" = 8
  dimension "d501" = 8
  dimension "d502" = 8
  dimension "d503" = 8
  measures "d489" diameter of A31
  measures "d490" diameter of A32
  measures "d491" diameter of A33
  measures "d492" diameter of A34
  measures "d493" diameter of A35
  measures "d494" diameter of A36
  measures "d495" diameter of A37
  measures "d496" diameter of A38
  measures "d497" diameter of A39
  measures "d498" diameter of A40
  measures "d499" diameter of A41
  measures "d500" diameter of A42
  measures "d501" diameter of A43
  measures "d502" diameter of A44
  measures "d503" diameter of A45
extrude "Extrude65" cut sketch "Sketch101" against normal blind 10 contours A31 | A32 | A33 | A34 | A35 | A36 | A37 | A38 | A39 | A40 | A41 | A42 | A43 | A44 | A45 bodies 2
sketch "Sketch102" plane through (-422.6941, 0, 0) normal (1, 0, 0) x (0, 1, 0)
  arc A0 (0, 130.6014) -> (0, 125.6014) centre (0, 128.1014) ccw
  line L0 (0, 130.6014) -> (0, 150.6014)
  arc A1 (0, 155.6014) -> (0, 150.6014) centre (0, 153.1014) ccw
  line L1 (0, 155.6014) -> (10, 155.6014)
  line L2 (10, 155.6014) -> (10, 273.6512)
  line L3 (10, 273.6512) -> (-30, 273.6512)
  line L4 (-30, 273.6512) -> (-30, 263.6512)
  arc A2 (-35, 263.6512) -> (-30, 263.6512) centre (-32.5, 263.6512) ccw
  line L5 (-35, 263.6512) -> (-55, 263.6512)
  arc A3 (-60, 263.6512) -> (-55, 263.6512) centre (-57.5, 263.6512) ccw
  line L6 (-60, 263.6512) -> (-60, 273.6512)
  line L7 (-60, 273.6512) -> (-100, 273.6512)
  line L8 (-100, 273.6512) -> (-100, -256.3488)
  line L9 (-100, -256.3488) -> (-60, -256.3488)
  line L10 (-60, -256.3488) -> (-60, -246.3488)
  arc A4 (-55, -246.3488) -> (-60, -246.3488) centre (-57.5, -246.3488) ccw
  line L11 (-55, -246.3488) -> (-35, -246.3488)
  arc A5 (-30, -246.3488) -> (-35, -246.3488) centre (-32.5, -246.3488) ccw
  line L12 (-30, -246.3488) -> (-30, -256.3488)
  line L13 (-30, -256.3488) -> (10, -256.3488)
  line L14 (10, -256.3488) -> (10, -149.3986)
  line L15 (10, -149.3986) -> (0, -149.3986)
  arc A6 (0, -144.3986) -> (0, -149.3986) centre (0, -146.8986) ccw
  line L16 (0, -144.3986) -> (0, -124.3986)
  arc A7 (0, -119.3986) -> (0, -124.3986) centre (0, -121.8986) ccw
  line L17 (0, -119.3986) -> (10, -119.3986)
  line L18 (10, -119.3986) -> (10, -11.8986)
  line L19 (10, -11.8986) -> (0, -11.8986)
  arc A8 (0, -6.8986) -> (0, -11.8986) centre (0, -9.3986) ccw
  line L20 (0, -6.8986) -> (0, 13.1014)
  arc A9 (0, 18.1014) -> (0, 13.1014) centre (0, 15.6014) ccw
  line L21 (0, 18.1014) -> (10, 18.1014)
  line L22 (10, 18.1014) -> (10, 125.6014)
  line L23 (10, 125.6014) -> (0, 125.6014)
  circle A10 centre (-25, -180) radius 4
  circle A11 centre (-50, 175) radius 4
  circle A12 centre (-25, 170) radius 4
  circle A13 centre (-50, -175) radius 4
  circle A14 centre (-75, 180) radius 4
  circle A15 centre (-75, -170) radius 4
  circle A16 centre (-75, 160) radius 4
  circle A17 centre (-50, 155) radius 4
  circle A18 centre (-25, 150) radius 4
  circle A19 centre (-75, 140) radius 4
  circle A20 centre (-50, 134) radius 4
  circle A21 centre (-25, 130) radius 4
  circle A22 centre (-75, 120) radius 4
  circle A23 centre (-50, 115) radius 4
  circle A24 centre (-25, 110) radius 4
  circle A25 centre (-75, 100) radius 4
  circle A26 centre (-50, 95) radius 4
  circle A27 centre (-25, 90) radius 4
  circle A28 centre (-75, 80) radius 4
  circle A29 centre (-50, 75) radius 4
  circle A30 centre (-25, 70) radius 4
  dimension "d506" = 20
  dimension "d507" = 8
  dimension "d508" = 8
  dimension "d509" = 8
  dimension "d510" = 8
  dimension "d511" = 8
  dimension "d512" = 8
  dimension "d513" = 8
  dimension "d514" = 8
  dimension "d515" = 8
  dimension "d516" = 8
  dimension "d517" = 8
  dimension "d518" = 8
  dimension "d519" = 8
  dimension "d520" = 8
  dimension "d521" = 8
  measures "d506" distance of A14.centre A16.centre
  measures "d507" diameter of A16
  measures "d508" diameter of A17
  measures "d509" diameter of A18
  measures "d510" diameter of A19
  measures "d511" diameter of A20
  measures "d512" diameter of A21
  measures "d513" diameter of A22
  measures "d514" diameter of A23
  measures "d515" diameter of A24
  measures "d516" diameter of A25
  measures "d517" diameter of A26
  measures "d518" diameter of A27
  measures "d519" diameter of A28
  measures "d520" diameter of A29
  measures "d521" diameter of A30
extrude "Extrude66" cut sketch "Sketch102" against normal blind 10 contours A16 | A17 | A18 | A19 | A20 | A21 | A22 | A23 | A24 | A25 | A26 | A27 | A28 | A29 | A30 bodies 3
sketch "Sketch103" plane through (-422.6941, 0, 0) normal (1, 0, 0) x (0, 1, 0)
  circle A0 centre (-75, 80) radius 4
  circle A1 centre (-25, 110) radius 4
  circle A2 centre (-50, 134) radius 4
  circle A3 centre (-75, 160) radius 4
  circle A4 centre (-75, 140) radius 4
  circle A5 centre (-50, 115) radius 4
  circle A6 centre (-25, 90) radius 4
  circle A7 centre (-50, 75) radius 4
  circle A8 centre (-75, 100) radius 4
  circle A9 centre (-25, 130) radius 4
  circle A10 centre (-50, 155) radius 4
  circle A11 centre (-25, 150) radius 4
  circle A12 centre (-75, 120) radius 4
  circle A13 centre (-50, 95) radius 4
  circle A14 centre (-25, 70) radius 4
  arc A15 (0, 130.6014) -> (0, 125.6014) centre (0, 128.1014) ccw
  line L0 (0, 130.6014) -> (0, 150.6014)
  arc A16 (0, 155.6014) -> (0, 150.6014) centre (0, 153.1014) ccw
  line L1 (0, 155.6014) -> (10, 155.6014)
  line L2 (10, 155.6014) -> (10, 273.6512)
  line L3 (10, 273.6512) -> (-30, 273.6512)
  line L4 (-30, 273.6512) -> (-30, 263.6512)
  arc A17 (-35, 263.6512) -> (-30, 263.6512) centre (-32.5, 263.6512) ccw
  line L5 (-35, 263.6512) -> (-55, 263.6512)
  arc A18 (-60, 263.6512) -> (-55, 263.6512) centre (-57.5, 263.6512) ccw
  line L6 (-60, 263.6512) -> (-60, 273.6512)
  line L7 (-60, 273.6512) -> (-100, 273.6512)
  line L8 (-100, 273.6512) -> (-100, -256.3488)
  line L9 (-100, -256.3488) -> (-60, -256.3488)
  line L10 (-60, -256.3488) -> (-60, -246.3488)
  arc A19 (-55, -246.3488) -> (-60, -246.3488) centre (-57.5, -246.3488) ccw
  line L11 (-55, -246.3488) -> (-35, -246.3488)
  arc A20 (-30, -246.3488) -> (-35, -246.3488) centre (-32.5, -246.3488) ccw
  line L12 (-30, -246.3488) -> (-30, -256.3488)
  line L13 (-30, -256.3488) -> (10, -256.3488)
  line L14 (10, -256.3488) -> (10, -149.3986)
  line L15 (10, -149.3986) -> (0, -149.3986)
  arc A21 (0, -144.3986) -> (0, -149.3986) centre (0, -146.8986) ccw
  line L16 (0, -144.3986) -> (0, -124.3986)
  arc A22 (0, -119.3986) -> (0, -124.3986) centre (0, -121.8986) ccw
  line L17 (0, -119.3986) -> (10, -119.3986)
  line L18 (10, -119.3986) -> (10, -11.8986)
  line L19 (10, -11.8986) -> (0, -11.8986)
  arc A23 (0, -6.8986) -> (0, -11.8986) centre (0, -9.3986) ccw
  line L20 (0, -6.8986) -> (0, 13.1014)
  arc A24 (0, 18.1014) -> (0, 13.1014) centre (0, 15.6014) ccw
  line L21 (0, 18.1014) -> (10, 18.1014)
  line L22 (10, 18.1014) -> (10, 125.6014)
  line L23 (10, 125.6014) -> (0, 125.6014)
  circle A25 centre (-25, -180) radius 4
  circle A26 centre (-50, 175) radius 4
  circle A27 centre (-25, 170) radius 4
  circle A28 centre (-50, -175) radius 4
  circle A29 centre (-75, 180) radius 4
  circle A30 centre (-75, -170) radius 4
  circle A31 centre (-75, -150) radius 4
  circle A32 centre (-50, -155) radius 4
  circle A33 centre (-25, -160) radius 4
  circle A34 centre (-75, -130) radius 4
  circle A35 centre (-50, -135) radius 4
  circle A36 centre (-25, -140) radius 4
  circle A37 centre (-75, -110) radius 4
  circle A38 centre (-50, -115) radius 4
  circle A39 centre (-25, -120) radius 4
  circle A40 centre (-75, -90) radius 4
  circle A41 centre (-50, -95) radius 4
  circle A42 centre (-25, -100) radius 4
  circle A43 centre (-75, -70) radius 4
  circle A44 centre (-50, -75) radius 4
  circle A45 centre (-25, -80) radius 4
  dimension "d524" = 8
  dimension "d525" = 8
  dimension "d526" = 8
  dimension "d527" = 8
  dimension "d528" = 8
  dimension "d530" = 8
  dimension "d531" = 8
  dimension "d532" = 8
  dimension "d533" = 8
  dimension "d534" = 8
  dimension "d535" = 8
  dimension "d536" = 8
  dimension "d537" = 8
  dimension "d538" = 8
  dimension "d539" = 8
  measures "d524" diameter of A31
  measures "d525" diameter of A32
  measures "d526" diameter of A33
  measures "d527" diameter of A34
  measures "d528" diameter of A35
  measures "d530" diameter of A36
  measures "d531" diameter of A37
  measures "d532" diameter of A38
  measures "d533" diameter of A39
  measures "d534" diameter of A40
  measures "d535" diameter of A41
  measures "d536" diameter of A42
  measures "d537" diameter of A43
  measures "d538" diameter of A44
  measures "d539" diameter of A45
extrude "Extrude67" cut sketch "Sketch103" against normal blind 10 contours A31 | A32 | A33 | A34 | A35 | A36 | A37 | A38 | A39 | A40 | A41 | A42 | A43 | A44 | A45 bodies 3
move_body "Move25" bodies 30 to x (1, 0, 0) y (0, 1, 0) z (0, 0, 1) at (0, -38, 0)
sketch "Sketch104" plane through (0, -41, 0) normal (0, -1, 0) x (1, 0, 0)
  circle A0 centre (-282.6941, 15.6014) radius 82.5
  line L0 (-412.6941, -83.8986) -> (-392.6941, -103.8986)
  line L1 (-392.6941, -103.8986) -> (-172.6941, -103.8986)
  line L2 (-172.6941, -103.8986) -> (-152.6941, -83.8986)
  line L3 (-152.6941, -83.8986) -> (-152.6941, 116.1014)
  line L4 (-152.6941, 116.1014) -> (-172.6941, 136.1014)
  line L5 (-172.6941, 136.1014) -> (-392.6941, 136.1014)
  line L6 (-392.6941, 136.1014) -> (-412.6941, 116.1014)
  line L7 (-412.6941, 116.1014) -> (-412.6941, -83.8986)
  line L8 (-352.6941, 131.1014) -> (-332.6941, 131.1014)
  line L9 (-332.6941, 131.1014) -> (-332.6941, 121.1014)
  line L10 (-332.6941, 121.1014) -> (-352.6941, 121.1014)
  line L11 (-352.6941, 121.1014) -> (-352.6941, 131.1014)
  line L12 (-232.6941, 131.1014) -> (-212.6941, 131.1014)
  line L13 (-212.6941, 131.1014) -> (-212.6941, 121.1014)
  line L14 (-212.6941, 121.1014) -> (-232.6941, 121.1014)
  line L15 (-232.6941, 121.1014) -> (-232.6941, 131.1014)
  dimension "d542" = 20
  dimension "d543" = 10
  dimension "d544" = 20
  dimension "d545" = 10
  constraint horizontal L8
  constraint vertical L9
  constraint horizontal L10
  constraint vertical L11
  constraint horizontal L12
  constraint vertical L13
  constraint horizontal L14
  constraint vertical L15
  measures "d542" distance of L8.start L8.end
  measures "d543" distance of L8.start L10.end
  measures "d544" distance of L12.start L12.end
  measures "d545" distance of L12.start L14.end
extrude "Extrude68" add sketch "Sketch104" along normal blind 10 separate body contours L8 L9 L10 L11 | L12 L13 L14 L15 makes body 31 at (-346.0274, -44.3333, 131.1014) makes body 32 at (-226.0274, -44.3333, 131.1014)
sketch "Sketch105" plane through (-212.6941, 0, 0) normal (1, 0, 0) x (0, 1, 0)
  line L0 (-41, 121.1014) -> (-41, 131.1014)
  line L1 (-41, 131.1014) -> (-51, 131.1014)
  line L2 (-51, 131.1014) -> (-51, 121.1014)
  line L3 (-51, 121.1014) -> (-41, 121.1014)
  circle A0 centre (-46, 126.1014) radius 3
  dimension "d550" = 6
  measures "d550" diameter of A0
extrude "Extrude69" add sketch "Sketch105" against normal up to surface (140 mm away) separate body contours A0 makes body 33